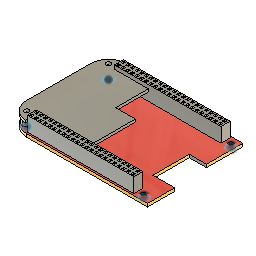
Proyektor New v3 (Autodesk Fusion 360 design; units mm, degrees)
Autodesk Fusion 360 part; units mm, degrees
sketch "Sketch1" plane through (0, 0, 0) normal (0, 0, 1) x (1, 0, 0)
  line L0 (35.75, 27.5) -> (-28.25, 27.5)
  line L1 (-38.25, 17.5) -> (-38.25, -17.5)
  line L2 (-28.25, -27.5) -> (38.25, -27.5)
  line L3 (38.25, -27.5) -> (38.25, -12.5)
  line L4 (35.75, 25.7026) -> (-34.8231, -25.0362) construction
  line L5 (-34.8231, 25.0362) -> (38.25, -27.5) construction
  line L6 (38.25, -27.5) -> (38.25, -12.5)
  line L7 (38.25, -12.5) -> (26.25, -12.5)
  line L8 (26.25, -12.5) -> (26.25, 7.5)
  line L9 (26.25, 7.5) -> (35.75, 7.5)
  line L10 (35.75, 7.5) -> (35.75, 27.5)
  arc A0 (-28.25, 27.5) -> (-38.25, 17.5) centre (-28.25, 17.5) ccw
  arc A1 (-38.25, -17.5) -> (-28.25, -27.5) centre (-28.25, -17.5) ccw
  dimension "d3" = 15
  dimension "d4" = 12
  dimension "d5" = 20
  dimension "d6" = 9.5
  dimension "d7" = 10
  constraint horizontal L0
  constraint perpendicular L0 L1
  constraint parallel L0 L2
  constraint parallel L1 L3
  constraint coincident L4 origin
  constraint coincident L5 origin
  constraint perpendicular L2 L6
  constraint perpendicular L3 L7
  constraint perpendicular L7 L8
  constraint perpendicular L3 L9
  constraint perpendicular L0 L10
  constraint tangent L0 A0
  constraint tangent L1 A0
  constraint tangent L1 A1
  constraint tangent L2 A1
  constraint equal A0 A1
  constraint coincident L10 L4.start
  constraint coincident A1 L4.end
  constraint coincident A0 L5.start
  measures "d3" distance of L2.end L3.end
  measures "d4" distance of L3.end L7.end
  measures "d5" distance of L7.end L8.end
  measures "d6" distance of L8.end L9.end
  measures "d7" radius of A0
extrude "Extrude1" add sketch "Sketch1" along normal blind 1.67 makes body 1
sketch "Sketch2" plane through (0, 0, 1.67) normal (0, 0, 1) x (-1, 0, 0)
  arc A0 (38.25, 17.5) -> (28.25, 27.5) centre (28.25, 17.5) ccw
  line L0 (28.25, 27.5) -> (-38.25, 27.5)
  line L1 (-38.25, 27.5) -> (-38.25, 12.5)
  line L2 (-38.25, 12.5) -> (-26.25, 12.5)
  line L3 (-26.25, 12.5) -> (-26.25, -7.5)
  line L4 (-26.25, -7.5) -> (-35.75, -7.5)
  line L5 (-35.75, -7.5) -> (-35.75, -27.5)
  line L6 (-35.75, -27.5) -> (28.25, -27.5)
  arc A1 (28.25, -27.5) -> (38.25, -17.5) centre (28.25, -17.5) ccw
  line L7 (38.25, -17.5) -> (38.25, 17.5)
  line L8 (-29.75, -26.5) -> (29.05, -26.5)
  line L9 (29.05, -26.5) -> (29.05, -21.5)
  line L10 (29.05, -21.5) -> (-29.75, -21.5)
  line L11 (-29.75, -21.5) -> (-29.75, -26.5)
  circle A2 centre (-32.75, -24) radius 1.25
  line L12 (-29.75, -24) -> (29.05, -24)
  line L13 (29.05, -24) -> (29.05, -26.5)
  line L14 (27.18, -24.65) -> (28.38, -24.65)
  line L15 (28.38, -24.65) -> (28.38, -25.85)
  line L16 (28.38, -25.85) -> (27.18, -25.85)
  line L17 (27.18, -25.85) -> (27.18, -24.65)
  line L18 (27.18, -24.65) -> (28.38, -25.85) construction
  line L19 (28.38, -24.65) -> (27.18, -25.85) construction
  line L20 (28.38, -22.15) -> (27.18, -22.15)
  line L21 (28.38, -23.35) -> (28.38, -22.15)
  line L22 (27.18, -22.15) -> (27.18, -23.35)
  line L23 (27.18, -23.35) -> (28.38, -23.35)
  line L24 (25.84, -25.85) -> (24.64, -25.85)
  line L25 (25.84, -24.65) -> (25.84, -25.85)
  line L26 (24.64, -25.85) -> (24.64, -24.65)
  line L27 (24.64, -24.65) -> (25.84, -24.65)
  line L28 (24.64, -23.35) -> (25.84, -23.35)
  line L29 (25.84, -23.35) -> (25.84, -22.15)
  line L30 (24.64, -22.15) -> (24.64, -23.35)
  line L31 (25.84, -22.15) -> (24.64, -22.15)
  line L32 (23.3, -25.85) -> (22.1, -25.85)
  line L33 (23.3, -24.65) -> (23.3, -25.85)
  line L34 (22.1, -25.85) -> (22.1, -24.65)
  line L35 (22.1, -24.65) -> (23.3, -24.65)
  line L36 (22.1, -23.35) -> (23.3, -23.35)
  line L37 (23.3, -23.35) -> (23.3, -22.15)
  line L38 (22.1, -22.15) -> (22.1, -23.35)
  line L39 (23.3, -22.15) -> (22.1, -22.15)
  line L40 (20.76, -25.85) -> (19.56, -25.85)
  line L41 (20.76, -24.65) -> (20.76, -25.85)
  line L42 (19.56, -25.85) -> (19.56, -24.65)
  line L43 (19.56, -24.65) -> (20.76, -24.65)
  line L44 (19.56, -23.35) -> (20.76, -23.35)
  line L45 (20.76, -23.35) -> (20.76, -22.15)
  line L46 (19.56, -22.15) -> (19.56, -23.35)
  line L47 (20.76, -22.15) -> (19.56, -22.15)
  line L48 (18.22, -25.85) -> (17.02, -25.85)
  line L49 (18.22, -24.65) -> (18.22, -25.85)
  line L50 (17.02, -25.85) -> (17.02, -24.65)
  line L51 (17.02, -24.65) -> (18.22, -24.65)
  line L52 (17.02, -23.35) -> (18.22, -23.35)
  line L53 (18.22, -23.35) -> (18.22, -22.15)
  line L54 (17.02, -22.15) -> (17.02, -23.35)
  line L55 (18.22, -22.15) -> (17.02, -22.15)
  line L56 (15.68, -25.85) -> (14.48, -25.85)
  line L57 (15.68, -24.65) -> (15.68, -25.85)
  line L58 (14.48, -25.85) -> (14.48, -24.65)
  line L59 (14.48, -24.65) -> (15.68, -24.65)
  line L60 (14.48, -23.35) -> (15.68, -23.35)
  line L61 (15.68, -23.35) -> (15.68, -22.15)
  line L62 (14.48, -22.15) -> (14.48, -23.35)
  line L63 (15.68, -22.15) -> (14.48, -22.15)
  line L64 (13.14, -25.85) -> (11.94, -25.85)
  line L65 (13.14, -24.65) -> (13.14, -25.85)
  line L66 (11.94, -25.85) -> (11.94, -24.65)
  line L67 (11.94, -24.65) -> (13.14, -24.65)
  line L68 (11.94, -23.35) -> (13.14, -23.35)
  line L69 (13.14, -23.35) -> (13.14, -22.15)
  line L70 (11.94, -22.15) -> (11.94, -23.35)
  line L71 (13.14, -22.15) -> (11.94, -22.15)
  line L72 (10.6, -25.85) -> (9.4, -25.85)
  line L73 (10.6, -24.65) -> (10.6, -25.85)
  line L74 (9.4, -25.85) -> (9.4, -24.65)
  line L75 (9.4, -24.65) -> (10.6, -24.65)
  line L76 (9.4, -23.35) -> (10.6, -23.35)
  line L77 (10.6, -23.35) -> (10.6, -22.15)
  line L78 (9.4, -22.15) -> (9.4, -23.35)
  line L79 (10.6, -22.15) -> (9.4, -22.15)
  line L80 (8.06, -25.85) -> (6.86, -25.85)
  line L81 (8.06, -24.65) -> (8.06, -25.85)
  line L82 (6.86, -25.85) -> (6.86, -24.65)
  line L83 (6.86, -24.65) -> (8.06, -24.65)
  line L84 (6.86, -23.35) -> (8.06, -23.35)
  line L85 (8.06, -23.35) -> (8.06, -22.15)
  line L86 (6.86, -22.15) -> (6.86, -23.35)
  line L87 (8.06, -22.15) -> (6.86, -22.15)
  line L88 (5.52, -25.85) -> (4.32, -25.85)
  line L89 (5.52, -24.65) -> (5.52, -25.85)
  line L90 (4.32, -25.85) -> (4.32, -24.65)
  line L91 (4.32, -24.65) -> (5.52, -24.65)
  line L92 (4.32, -23.35) -> (5.52, -23.35)
  line L93 (5.52, -23.35) -> (5.52, -22.15)
  line L94 (4.32, -22.15) -> (4.32, -23.35)
  line L95 (5.52, -22.15) -> (4.32, -22.15)
  line L96 (2.98, -25.85) -> (1.78, -25.85)
  line L97 (2.98, -24.65) -> (2.98, -25.85)
  line L98 (1.78, -25.85) -> (1.78, -24.65)
  line L99 (1.78, -24.65) -> (2.98, -24.65)
  line L100 (1.78, -23.35) -> (2.98, -23.35)
  line L101 (2.98, -23.35) -> (2.98, -22.15)
  line L102 (1.78, -22.15) -> (1.78, -23.35)
  line L103 (2.98, -22.15) -> (1.78, -22.15)
  line L104 (0.44, -25.85) -> (-0.76, -25.85)
  line L105 (0.44, -24.65) -> (0.44, -25.85)
  line L106 (-0.76, -25.85) -> (-0.76, -24.65)
  line L107 (-0.76, -24.65) -> (0.44, -24.65)
  line L108 (-0.76, -23.35) -> (0.44, -23.35)
  line L109 (0.44, -23.35) -> (0.44, -22.15)
  line L110 (-0.76, -22.15) -> (-0.76, -23.35)
  line L111 (0.44, -22.15) -> (-0.76, -22.15)
  line L112 (-2.1, -25.85) -> (-3.3, -25.85)
  line L113 (-2.1, -24.65) -> (-2.1, -25.85)
  line L114 (-3.3, -25.85) -> (-3.3, -24.65)
  line L115 (-3.3, -24.65) -> (-2.1, -24.65)
  line L116 (-3.3, -23.35) -> (-2.1, -23.35)
  line L117 (-2.1, -23.35) -> (-2.1, -22.15)
  line L118 (-3.3, -22.15) -> (-3.3, -23.35)
  line L119 (-2.1, -22.15) -> (-3.3, -22.15)
  line L120 (-4.64, -25.85) -> (-5.84, -25.85)
  line L121 (-4.64, -24.65) -> (-4.64, -25.85)
  line L122 (-5.84, -25.85) -> (-5.84, -24.65)
  line L123 (-5.84, -24.65) -> (-4.64, -24.65)
  line L124 (-5.84, -23.35) -> (-4.64, -23.35)
  line L125 (-4.64, -23.35) -> (-4.64, -22.15)
  line L126 (-5.84, -22.15) -> (-5.84, -23.35)
  line L127 (-4.64, -22.15) -> (-5.84, -22.15)
  line L128 (-7.18, -25.85) -> (-8.38, -25.85)
  line L129 (-7.18, -24.65) -> (-7.18, -25.85)
  line L130 (-8.38, -25.85) -> (-8.38, -24.65)
  line L131 (-8.38, -24.65) -> (-7.18, -24.65)
  line L132 (-8.38, -23.35) -> (-7.18, -23.35)
  line L133 (-7.18, -23.35) -> (-7.18, -22.15)
  line L134 (-8.38, -22.15) -> (-8.38, -23.35)
  line L135 (-7.18, -22.15) -> (-8.38, -22.15)
  line L136 (-9.72, -25.85) -> (-10.92, -25.85)
  line L137 (-9.72, -24.65) -> (-9.72, -25.85)
  line L138 (-10.92, -25.85) -> (-10.92, -24.65)
  line L139 (-10.92, -24.65) -> (-9.72, -24.65)
  line L140 (-10.92, -23.35) -> (-9.72, -23.35)
  line L141 (-9.72, -23.35) -> (-9.72, -22.15)
  line L142 (-10.92, -22.15) -> (-10.92, -23.35)
  line L143 (-9.72, -22.15) -> (-10.92, -22.15)
  line L144 (-12.26, -25.85) -> (-13.46, -25.85)
  line L145 (-12.26, -24.65) -> (-12.26, -25.85)
  line L146 (-13.46, -25.85) -> (-13.46, -24.65)
  line L147 (-13.46, -24.65) -> (-12.26, -24.65)
  line L148 (-13.46, -23.35) -> (-12.26, -23.35)
  line L149 (-12.26, -23.35) -> (-12.26, -22.15)
  line L150 (-13.46, -22.15) -> (-13.46, -23.35)
  line L151 (-12.26, -22.15) -> (-13.46, -22.15)
  line L152 (-14.8, -25.85) -> (-16, -25.85)
  line L153 (-14.8, -24.65) -> (-14.8, -25.85)
  line L154 (-16, -25.85) -> (-16, -24.65)
  line L155 (-16, -24.65) -> (-14.8, -24.65)
  line L156 (-16, -23.35) -> (-14.8, -23.35)
  line L157 (-14.8, -23.35) -> (-14.8, -22.15)
  line L158 (-16, -22.15) -> (-16, -23.35)
  line L159 (-14.8, -22.15) -> (-16, -22.15)
  line L160 (-17.34, -25.85) -> (-18.54, -25.85)
  line L161 (-17.34, -24.65) -> (-17.34, -25.85)
  line L162 (-18.54, -25.85) -> (-18.54, -24.65)
  line L163 (-18.54, -24.65) -> (-17.34, -24.65)
  line L164 (-18.54, -23.35) -> (-17.34, -23.35)
  line L165 (-17.34, -23.35) -> (-17.34, -22.15)
  line L166 (-18.54, -22.15) -> (-18.54, -23.35)
  line L167 (-17.34, -22.15) -> (-18.54, -22.15)
  line L168 (-19.88, -25.85) -> (-21.08, -25.85)
  line L169 (-19.88, -24.65) -> (-19.88, -25.85)
  line L170 (-21.08, -25.85) -> (-21.08, -24.65)
  line L171 (-21.08, -24.65) -> (-19.88, -24.65)
  line L172 (-21.08, -23.35) -> (-19.88, -23.35)
  line L173 (-19.88, -23.35) -> (-19.88, -22.15)
  line L174 (-21.08, -22.15) -> (-21.08, -23.35)
  line L175 (-19.88, -22.15) -> (-21.08, -22.15)
  line L176 (-22.42, -25.85) -> (-23.62, -25.85)
  line L177 (-22.42, -24.65) -> (-22.42, -25.85)
  line L178 (-23.62, -25.85) -> (-23.62, -24.65)
  line L179 (-23.62, -24.65) -> (-22.42, -24.65)
  line L180 (-23.62, -23.35) -> (-22.42, -23.35)
  line L181 (-22.42, -23.35) -> (-22.42, -22.15)
  line L182 (-23.62, -22.15) -> (-23.62, -23.35)
  line L183 (-22.42, -22.15) -> (-23.62, -22.15)
  line L184 (-24.96, -25.85) -> (-26.16, -25.85)
  line L185 (-24.96, -24.65) -> (-24.96, -25.85)
  line L186 (-26.16, -25.85) -> (-26.16, -24.65)
  line L187 (-26.16, -24.65) -> (-24.96, -24.65)
  line L188 (-26.16, -23.35) -> (-24.96, -23.35)
  line L189 (-24.96, -23.35) -> (-24.96, -22.15)
  line L190 (-26.16, -22.15) -> (-26.16, -23.35)
  line L191 (-24.96, -22.15) -> (-26.16, -22.15)
  line L192 (-27.5, -25.85) -> (-28.7, -25.85)
  line L193 (-27.5, -24.65) -> (-27.5, -25.85)
  line L194 (-28.7, -25.85) -> (-28.7, -24.65)
  line L195 (-28.7, -24.65) -> (-27.5, -24.65)
  line L196 (-28.7, -23.35) -> (-27.5, -23.35)
  line L197 (-27.5, -23.35) -> (-27.5, -22.15)
  line L198 (-28.7, -22.15) -> (-28.7, -23.35)
  line L199 (-27.5, -22.15) -> (-28.7, -22.15)
  circle A3 centre (33.25, -22.5) radius 1.25
  arc A4 (29.1, -27.4538) -> (38.24, -17.5) centre (28.25, -17.5) ccw
  line L200 (38.24, -17.5) -> (38.24, 17.5)
  arc A5 (38.24, 17.5) -> (29.1, 27.4538) centre (28.25, 17.5) ccw
  line L201 (29.1, -26.5) -> (29.1, -21.45)
  line L202 (29.1, -21.45) -> (10.24, -21.45)
  line L203 (29.1, -26.5) -> (29.1, -27.4538)
  line L204 (10.24, -21.45) -> (10.24, -3.45)
  line L205 (10.24, -3.45) -> (-0.56, -3.45)
  circle A6 centre (33.25, 22.5) radius 1.25
  line L206 (-28.7, 23.35) -> (-27.5, 23.35)
  line L207 (29.05, 21.5) -> (-29.75, 21.5)
  line L208 (29.1, 21.45) -> (-0.56, 21.45)
  line L209 (-29.75, 21.5) -> (-29.75, 26.5)
  line L210 (-22.42, 25.85) -> (-23.62, 25.85)
  line L211 (-19.88, 24.65) -> (-19.88, 25.85)
  line L212 (-21.08, 23.35) -> (-19.88, 23.35)
  line L213 (-23.62, 23.35) -> (-22.42, 23.35)
  line L214 (-24.96, 23.35) -> (-24.96, 22.15)
  line L215 (-27.5, 25.85) -> (-28.7, 25.85)
  line L216 (-22.42, 23.35) -> (-22.42, 22.15)
  line L217 (-29.75, 26.5) -> (29.05, 26.5)
  line L218 (-19.88, 25.85) -> (-21.08, 25.85)
  line L219 (-24.96, 24.65) -> (-24.96, 25.85)
  line L220 (-21.08, 22.15) -> (-21.08, 23.35)
  line L221 (-28.7, 24.65) -> (-27.5, 24.65)
  line L222 (-28.7, 22.15) -> (-28.7, 23.35)
  line L223 (-26.16, 25.85) -> (-26.16, 24.65)
  line L224 (-28.7, 25.85) -> (-28.7, 24.65)
  line L225 (-27.5, 23.35) -> (-27.5, 22.15)
  line L226 (-23.62, 25.85) -> (-23.62, 24.65)
  line L227 (-19.88, 23.35) -> (-19.88, 22.15)
  line L228 (-22.42, 22.15) -> (-23.62, 22.15)
  line L229 (-24.96, 22.15) -> (-26.16, 22.15)
  line L230 (-23.62, 24.65) -> (-22.42, 24.65)
  line L231 (-26.16, 24.65) -> (-24.96, 24.65)
  line L232 (-23.62, 22.15) -> (-23.62, 23.35)
  line L233 (-22.42, 24.65) -> (-22.42, 25.85)
  line L234 (-21.08, 24.65) -> (-19.88, 24.65)
  line L235 (-19.88, 22.15) -> (-21.08, 22.15)
  line L236 (-26.16, 22.15) -> (-26.16, 23.35)
  line L237 (-21.08, 25.85) -> (-21.08, 24.65)
  line L238 (-27.5, 24.65) -> (-27.5, 25.85)
  line L239 (-26.16, 23.35) -> (-24.96, 23.35)
  line L240 (-24.96, 25.85) -> (-26.16, 25.85)
  line L241 (-27.5, 22.15) -> (-28.7, 22.15)
  circle A7 centre (-32.75, 24) radius 1.25
  line L242 (-14.8, 23.35) -> (-14.8, 22.15)
  line L243 (-10.92, 23.35) -> (-9.72, 23.35)
  line L244 (-13.46, 24.65) -> (-12.26, 24.65)
  line L245 (-10.92, 25.85) -> (-10.92, 24.65)
  line L246 (-14.8, 24.65) -> (-14.8, 25.85)
  line L247 (8.06, 25.85) -> (6.86, 25.85)
  line L248 (-12.26, 23.35) -> (-12.26, 22.15)
  line L249 (-10.92, 24.65) -> (-9.72, 24.65)
  line L250 (-9.72, 23.35) -> (-9.72, 22.15)
  line L251 (-16, 23.35) -> (-14.8, 23.35)
  line L252 (-12.26, 25.85) -> (-13.46, 25.85)
  line L253 (-16, 24.65) -> (-14.8, 24.65)
  line L254 (-13.46, 25.85) -> (-13.46, 24.65)
  line L255 (-12.26, 24.65) -> (-12.26, 25.85)
  line L256 (-9.72, 24.65) -> (-9.72, 25.85)
  line L257 (1.78, 23.35) -> (2.98, 23.35)
  line L258 (-13.46, 23.35) -> (-12.26, 23.35)
  line L259 (-10.92, 22.15) -> (-10.92, 23.35)
  line L260 (-16, 22.15) -> (-16, 23.35)
  line L261 (-16, 25.85) -> (-16, 24.65)
  line L262 (-13.46, 22.15) -> (-13.46, 23.35)
  line L263 (-14.8, 25.85) -> (-16, 25.85)
  line L264 (-8.38, 25.85) -> (-8.38, 24.65)
  line L265 (1.78, 22.15) -> (1.78, 23.35)
  line L266 (-3.3, 25.85) -> (-3.3, 24.65)
  line L267 (-0.76, 22.15) -> (-0.76, 23.35)
  line L268 (22.1, 24.65) -> (23.3, 24.65)
  line L269 (20.76, 23.35) -> (20.76, 22.15)
  line L270 (28.38, 23.35) -> (28.38, 22.15)
  line L271 (9.4, 22.15) -> (9.4, 23.35)
  line L272 (10.6, 23.35) -> (10.6, 22.15)
  line L273 (22.1, 23.35) -> (23.3, 23.35)
  line L274 (23.3, 23.35) -> (23.3, 22.15)
  line L275 (9.4, 25.85) -> (9.4, 24.65)
  line L276 (25.84, 24.65) -> (25.84, 25.85)
  line L277 (25.84, 25.85) -> (24.64, 25.85)
  line L278 (-8.38, 24.65) -> (-7.18, 24.65)
  line L279 (6.86, 22.15) -> (6.86, 23.35)
  line L280 (28.38, 24.65) -> (28.38, 25.85)
  line L281 (0.44, 25.85) -> (-0.76, 25.85)
  line L282 (24.64, 22.15) -> (24.64, 23.35)
  line L283 (4.32, 22.15) -> (4.32, 23.35)
  line L284 (22.1, 25.85) -> (22.1, 24.65)
  line L285 (1.78, 25.85) -> (1.78, 24.65)
  line L286 (6.86, 25.85) -> (6.86, 24.65)
  line L287 (4.32, 25.85) -> (4.32, 24.65)
  line L288 (-8.38, 22.15) -> (-8.38, 23.35)
  line L289 (24.64, 24.65) -> (25.84, 24.65)
  line L290 (19.56, 22.15) -> (19.56, 23.35)
  line L291 (20.76, 25.85) -> (19.56, 25.85)
  line L292 (27.18, 22.15) -> (27.18, 23.35)
  line L293 (-9.72, 25.85) -> (-10.92, 25.85)
  line L294 (19.56, 23.35) -> (20.76, 23.35)
  line L295 (-2.1, 24.65) -> (-2.1, 25.85)
  line L296 (28.38, 25.85) -> (27.18, 25.85)
  line L297 (-4.64, 25.85) -> (-5.84, 25.85)
  line L298 (-17.34, 25.85) -> (-18.54, 25.85)
  line L299 (22.1, 22.15) -> (22.1, 23.35)
  line L300 (27.18, 23.35) -> (28.38, 23.35)
  line L301 (25.84, 23.35) -> (25.84, 22.15)
  line L302 (9.4, 23.35) -> (10.6, 23.35)
  line L303 (-18.54, 23.35) -> (-17.34, 23.35)
  line L304 (10.6, 25.85) -> (9.4, 25.85)
  line L305 (-4.64, 23.35) -> (-4.64, 22.15)
  line L306 (-3.3, 23.35) -> (-2.1, 23.35)
  line L307 (2.98, 23.35) -> (2.98, 22.15)
  line L308 (2.98, 25.85) -> (1.78, 25.85)
  line L309 (-18.54, 25.85) -> (-18.54, 24.65)
  line L310 (-0.76, 23.35) -> (0.44, 23.35)
  line L311 (-2.1, 25.85) -> (-3.3, 25.85)
  line L312 (19.56, 24.65) -> (20.76, 24.65)
  line L313 (4.32, 24.65) -> (5.52, 24.65)
  line L314 (8.06, 24.65) -> (8.06, 25.85)
  line L315 (19.56, 25.85) -> (19.56, 24.65)
  line L316 (-4.64, 24.65) -> (-4.64, 25.85)
  line L317 (27.18, 24.65) -> (28.38, 24.65)
  line L318 (1.78, 24.65) -> (2.98, 24.65)
  line L319 (0.44, 24.65) -> (0.44, 25.85)
  line L320 (23.3, 25.85) -> (22.1, 25.85)
  line L321 (9.4, 24.65) -> (10.6, 24.65)
  line L322 (24.64, 25.85) -> (24.64, 24.65)
  line L323 (-0.76, 24.65) -> (0.44, 24.65)
  line L324 (-3.3, 24.65) -> (-2.1, 24.65)
  line L325 (-17.34, 23.35) -> (-17.34, 22.15)
  line L326 (-7.18, 25.85) -> (-8.38, 25.85)
  line L327 (-5.84, 24.65) -> (-4.64, 24.65)
  line L328 (23.3, 24.65) -> (23.3, 25.85)
  line L329 (27.18, 25.85) -> (27.18, 24.65)
  line L330 (5.52, 23.35) -> (5.52, 22.15)
  line L331 (-3.3, 22.15) -> (-3.3, 23.35)
  line L332 (6.86, 23.35) -> (8.06, 23.35)
  line L333 (0.44, 23.35) -> (0.44, 22.15)
  line L334 (-5.84, 22.15) -> (-5.84, 23.35)
  line L335 (10.6, 24.65) -> (10.6, 25.85)
  line L336 (24.64, 23.35) -> (25.84, 23.35)
  line L337 (-7.18, 23.35) -> (-7.18, 22.15)
  line L338 (-0.76, 25.85) -> (-0.76, 24.65)
  line L339 (5.52, 25.85) -> (4.32, 25.85)
  line L340 (20.76, 24.65) -> (20.76, 25.85)
  line L341 (-5.84, 25.85) -> (-5.84, 24.65)
  line L342 (-8.38, 23.35) -> (-7.18, 23.35)
  line L343 (2.98, 24.65) -> (2.98, 25.85)
  line L344 (-5.84, 23.35) -> (-4.64, 23.35)
  line L345 (-18.54, 22.15) -> (-18.54, 23.35)
  line L346 (-17.34, 24.65) -> (-17.34, 25.85)
  line L347 (-2.1, 23.35) -> (-2.1, 22.15)
  line L348 (-18.54, 24.65) -> (-17.34, 24.65)
  line L349 (-7.18, 24.65) -> (-7.18, 25.85)
  line L350 (14.48, 24.65) -> (15.68, 24.65)
  line L351 (5.52, 24.65) -> (5.52, 25.85)
  line L352 (11.94, 22.15) -> (11.94, 23.35)
  line L353 (17.02, 23.35) -> (18.22, 23.35)
  line L354 (15.68, 25.85) -> (14.48, 25.85)
  line L355 (13.14, 23.35) -> (13.14, 22.15)
  line L356 (18.22, 25.85) -> (17.02, 25.85)
  line L357 (14.48, 25.85) -> (14.48, 24.65)
  line L358 (17.02, 24.65) -> (18.22, 24.65)
  line L359 (17.02, 22.15) -> (17.02, 23.35)
  line L360 (18.22, 23.35) -> (18.22, 22.15)
  line L361 (4.32, 23.35) -> (5.52, 23.35)
  line L362 (14.48, 23.35) -> (15.68, 23.35)
  line L363 (13.14, 24.65) -> (13.14, 25.85)
  line L364 (11.94, 25.85) -> (11.94, 24.65)
  line L365 (18.22, 24.65) -> (18.22, 25.85)
  line L366 (14.48, 22.15) -> (14.48, 23.35)
  line L367 (15.68, 23.35) -> (15.68, 22.15)
  line L368 (8.06, 23.35) -> (8.06, 22.15)
  line L369 (17.02, 25.85) -> (17.02, 24.65)
  line L370 (6.86, 24.65) -> (8.06, 24.65)
  line L371 (13.14, 25.85) -> (11.94, 25.85)
  line L372 (11.94, 23.35) -> (13.14, 23.35)
  line L373 (11.94, 24.65) -> (13.14, 24.65)
  line L374 (15.68, 24.65) -> (15.68, 25.85)
  line L375 (28.38, 22.15) -> (27.18, 22.15)
  line L376 (25.84, 22.15) -> (24.64, 22.15)
  line L377 (23.3, 22.15) -> (22.1, 22.15)
  line L378 (20.76, 22.15) -> (19.56, 22.15)
  line L379 (18.22, 22.15) -> (17.02, 22.15)
  line L380 (15.68, 22.15) -> (14.48, 22.15)
  line L381 (13.14, 22.15) -> (11.94, 22.15)
  line L382 (10.6, 22.15) -> (9.4, 22.15)
  line L383 (8.06, 22.15) -> (6.86, 22.15)
  line L384 (5.52, 22.15) -> (4.32, 22.15)
  line L385 (2.98, 22.15) -> (1.78, 22.15)
  line L386 (0.44, 22.15) -> (-0.76, 22.15)
  line L387 (-2.1, 22.15) -> (-3.3, 22.15)
  line L388 (-4.64, 22.15) -> (-5.84, 22.15)
  line L389 (-7.18, 22.15) -> (-8.38, 22.15)
  line L390 (-9.72, 22.15) -> (-10.92, 22.15)
  line L391 (-12.26, 22.15) -> (-13.46, 22.15)
  line L392 (-14.8, 22.15) -> (-16, 22.15)
  line L393 (-17.34, 22.15) -> (-18.54, 22.15)
  line L394 (29.05, 21.5) -> (29.05, 26.5)
  line L395 (-0.56, -3.45) -> (-0.56, 21.45)
  line L396 (29.1, 21.45) -> (29.1, 27.4538)
  line L397 (27.58, 25.05) -> (27.98, 25.05)
  line L398 (27.98, 25.05) -> (27.98, 25.45)
  line L399 (27.98, 25.45) -> (27.58, 25.45)
  line L400 (27.58, 25.45) -> (27.58, 25.05)
  line L401 (29.05, 24) -> (27.6, 24)
  line L402 (27.98, 22.95) -> (27.98, 22.55)
  line L403 (27.58, 22.95) -> (27.98, 22.95)
  line L404 (27.58, 22.55) -> (27.58, 22.95)
  line L405 (27.98, 22.55) -> (27.58, 22.55)
  line L406 (25.04, 25.45) -> (25.04, 25.05)
  line L407 (25.44, 25.05) -> (25.44, 25.45)
  line L408 (25.04, 25.05) -> (25.44, 25.05)
  line L409 (25.44, 25.45) -> (25.04, 25.45)
  line L410 (25.04, 22.95) -> (25.44, 22.95)
  line L411 (25.44, 22.55) -> (25.04, 22.55)
  line L412 (25.44, 22.95) -> (25.44, 22.55)
  line L413 (25.04, 22.55) -> (25.04, 22.95)
  line L414 (22.5, 25.45) -> (22.5, 25.05)
  line L415 (22.9, 25.05) -> (22.9, 25.45)
  line L416 (22.5, 25.05) -> (22.9, 25.05)
  line L417 (22.9, 25.45) -> (22.5, 25.45)
  line L418 (22.5, 22.95) -> (22.9, 22.95)
  line L419 (22.9, 22.55) -> (22.5, 22.55)
  line L420 (22.9, 22.95) -> (22.9, 22.55)
  line L421 (22.5, 22.55) -> (22.5, 22.95)
  line L422 (19.96, 25.45) -> (19.96, 25.05)
  line L423 (20.36, 25.05) -> (20.36, 25.45)
  line L424 (19.96, 25.05) -> (20.36, 25.05)
  line L425 (20.36, 25.45) -> (19.96, 25.45)
  line L426 (19.96, 22.95) -> (20.36, 22.95)
  line L427 (20.36, 22.55) -> (19.96, 22.55)
  line L428 (20.36, 22.95) -> (20.36, 22.55)
  line L429 (19.96, 22.55) -> (19.96, 22.95)
  line L430 (17.42, 25.45) -> (17.42, 25.05)
  line L431 (17.82, 25.05) -> (17.82, 25.45)
  line L432 (17.42, 25.05) -> (17.82, 25.05)
  line L433 (17.82, 25.45) -> (17.42, 25.45)
  line L434 (17.42, 22.95) -> (17.82, 22.95)
  line L435 (17.82, 22.55) -> (17.42, 22.55)
  line L436 (17.82, 22.95) -> (17.82, 22.55)
  line L437 (17.42, 22.55) -> (17.42, 22.95)
  line L438 (14.88, 25.45) -> (14.88, 25.05)
  line L439 (15.28, 25.05) -> (15.28, 25.45)
  line L440 (14.88, 25.05) -> (15.28, 25.05)
  line L441 (15.28, 25.45) -> (14.88, 25.45)
  line L442 (14.88, 22.95) -> (15.28, 22.95)
  line L443 (15.28, 22.55) -> (14.88, 22.55)
  line L444 (15.28, 22.95) -> (15.28, 22.55)
  line L445 (14.88, 22.55) -> (14.88, 22.95)
  line L446 (12.34, 25.45) -> (12.34, 25.05)
  line L447 (12.74, 25.05) -> (12.74, 25.45)
  line L448 (12.34, 25.05) -> (12.74, 25.05)
  line L449 (12.74, 25.45) -> (12.34, 25.45)
  line L450 (12.34, 22.95) -> (12.74, 22.95)
  line L451 (12.74, 22.55) -> (12.34, 22.55)
  line L452 (12.74, 22.95) -> (12.74, 22.55)
  line L453 (12.34, 22.55) -> (12.34, 22.95)
  line L454 (9.8, 25.45) -> (9.8, 25.05)
  line L455 (10.2, 25.05) -> (10.2, 25.45)
  line L456 (9.8, 25.05) -> (10.2, 25.05)
  line L457 (10.2, 25.45) -> (9.8, 25.45)
  line L458 (9.8, 22.95) -> (10.2, 22.95)
  line L459 (10.2, 22.55) -> (9.8, 22.55)
  line L460 (10.2, 22.95) -> (10.2, 22.55)
  line L461 (9.8, 22.55) -> (9.8, 22.95)
  line L462 (7.26, 25.45) -> (7.26, 25.05)
  line L463 (7.66, 25.05) -> (7.66, 25.45)
  line L464 (7.26, 25.05) -> (7.66, 25.05)
  line L465 (7.66, 25.45) -> (7.26, 25.45)
  line L466 (7.26, 22.95) -> (7.66, 22.95)
  line L467 (7.66, 22.55) -> (7.26, 22.55)
  line L468 (7.66, 22.95) -> (7.66, 22.55)
  line L469 (7.26, 22.55) -> (7.26, 22.95)
  line L470 (4.72, 25.45) -> (4.72, 25.05)
  line L471 (5.12, 25.05) -> (5.12, 25.45)
  line L472 (4.72, 25.05) -> (5.12, 25.05)
  line L473 (5.12, 25.45) -> (4.72, 25.45)
  line L474 (4.72, 22.95) -> (5.12, 22.95)
  line L475 (5.12, 22.55) -> (4.72, 22.55)
  line L476 (5.12, 22.95) -> (5.12, 22.55)
  line L477 (4.72, 22.55) -> (4.72, 22.95)
  line L478 (2.18, 25.45) -> (2.18, 25.05)
  line L479 (2.58, 25.05) -> (2.58, 25.45)
  line L480 (2.18, 25.05) -> (2.58, 25.05)
  line L481 (2.58, 25.45) -> (2.18, 25.45)
  line L482 (2.18, 22.95) -> (2.58, 22.95)
  line L483 (2.58, 22.55) -> (2.18, 22.55)
  line L484 (2.58, 22.95) -> (2.58, 22.55)
  line L485 (2.18, 22.55) -> (2.18, 22.95)
  line L486 (-0.36, 25.45) -> (-0.36, 25.05)
  line L487 (0.04, 25.05) -> (0.04, 25.45)
  line L488 (-0.36, 25.05) -> (0.04, 25.05)
  line L489 (0.04, 25.45) -> (-0.36, 25.45)
  line L490 (-0.36, 22.95) -> (0.04, 22.95)
  line L491 (0.04, 22.55) -> (-0.36, 22.55)
  line L492 (0.04, 22.95) -> (0.04, 22.55)
  line L493 (-0.36, 22.55) -> (-0.36, 22.95)
  line L494 (-2.9, 25.45) -> (-2.9, 25.05)
  line L495 (-2.5, 25.05) -> (-2.5, 25.45)
  line L496 (-2.9, 25.05) -> (-2.5, 25.05)
  line L497 (-2.5, 25.45) -> (-2.9, 25.45)
  line L498 (-2.9, 22.95) -> (-2.5, 22.95)
  line L499 (-2.5, 22.55) -> (-2.9, 22.55)
  line L500 (-2.5, 22.95) -> (-2.5, 22.55)
  line L501 (-2.9, 22.55) -> (-2.9, 22.95)
  line L502 (-5.44, 25.45) -> (-5.44, 25.05)
  line L503 (-5.04, 25.05) -> (-5.04, 25.45)
  line L504 (-5.44, 25.05) -> (-5.04, 25.05)
  line L505 (-5.04, 25.45) -> (-5.44, 25.45)
  line L506 (-5.44, 22.95) -> (-5.04, 22.95)
  line L507 (-5.04, 22.55) -> (-5.44, 22.55)
  line L508 (-5.04, 22.95) -> (-5.04, 22.55)
  line L509 (-5.44, 22.55) -> (-5.44, 22.95)
  line L510 (-7.98, 25.45) -> (-7.98, 25.05)
  line L511 (-7.58, 25.05) -> (-7.58, 25.45)
  line L512 (-7.98, 25.05) -> (-7.58, 25.05)
  line L513 (-7.58, 25.45) -> (-7.98, 25.45)
  line L514 (-7.98, 22.95) -> (-7.58, 22.95)
  line L515 (-7.58, 22.55) -> (-7.98, 22.55)
  line L516 (-7.58, 22.95) -> (-7.58, 22.55)
  line L517 (-7.98, 22.55) -> (-7.98, 22.95)
  line L518 (-10.52, 25.45) -> (-10.52, 25.05)
  line L519 (-10.12, 25.05) -> (-10.12, 25.45)
  line L520 (-10.52, 25.05) -> (-10.12, 25.05)
  line L521 (-10.12, 25.45) -> (-10.52, 25.45)
  line L522 (-10.52, 22.95) -> (-10.12, 22.95)
  line L523 (-10.12, 22.55) -> (-10.52, 22.55)
  line L524 (-10.12, 22.95) -> (-10.12, 22.55)
  line L525 (-10.52, 22.55) -> (-10.52, 22.95)
  line L526 (-13.06, 25.45) -> (-13.06, 25.05)
  line L527 (-12.66, 25.05) -> (-12.66, 25.45)
  line L528 (-13.06, 25.05) -> (-12.66, 25.05)
  line L529 (-12.66, 25.45) -> (-13.06, 25.45)
  line L530 (-13.06, 22.95) -> (-12.66, 22.95)
  line L531 (-12.66, 22.55) -> (-13.06, 22.55)
  line L532 (-12.66, 22.95) -> (-12.66, 22.55)
  line L533 (-13.06, 22.55) -> (-13.06, 22.95)
  line L534 (-15.6, 25.45) -> (-15.6, 25.05)
  line L535 (-15.2, 25.05) -> (-15.2, 25.45)
  line L536 (-15.6, 25.05) -> (-15.2, 25.05)
  line L537 (-15.2, 25.45) -> (-15.6, 25.45)
  line L538 (-15.6, 22.95) -> (-15.2, 22.95)
  line L539 (-15.2, 22.55) -> (-15.6, 22.55)
  line L540 (-15.2, 22.95) -> (-15.2, 22.55)
  line L541 (-15.6, 22.55) -> (-15.6, 22.95)
  line L542 (-18.14, 25.45) -> (-18.14, 25.05)
  line L543 (-17.74, 25.05) -> (-17.74, 25.45)
  line L544 (-18.14, 25.05) -> (-17.74, 25.05)
  line L545 (-17.74, 25.45) -> (-18.14, 25.45)
  line L546 (-18.14, 22.95) -> (-17.74, 22.95)
  line L547 (-17.74, 22.55) -> (-18.14, 22.55)
  line L548 (-17.74, 22.95) -> (-17.74, 22.55)
  line L549 (-18.14, 22.55) -> (-18.14, 22.95)
  line L550 (-20.68, 25.45) -> (-20.68, 25.05)
  line L551 (-20.28, 25.05) -> (-20.28, 25.45)
  line L552 (-20.68, 25.05) -> (-20.28, 25.05)
  line L553 (-20.28, 25.45) -> (-20.68, 25.45)
  line L554 (-20.68, 22.95) -> (-20.28, 22.95)
  line L555 (-20.28, 22.55) -> (-20.68, 22.55)
  line L556 (-20.28, 22.95) -> (-20.28, 22.55)
  line L557 (-20.68, 22.55) -> (-20.68, 22.95)
  line L558 (-23.22, 25.45) -> (-23.22, 25.05)
  line L559 (-22.82, 25.05) -> (-22.82, 25.45)
  line L560 (-23.22, 25.05) -> (-22.82, 25.05)
  line L561 (-22.82, 25.45) -> (-23.22, 25.45)
  line L562 (-23.22, 22.95) -> (-22.82, 22.95)
  line L563 (-22.82, 22.55) -> (-23.22, 22.55)
  line L564 (-22.82, 22.95) -> (-22.82, 22.55)
  line L565 (-23.22, 22.55) -> (-23.22, 22.95)
  line L566 (-25.76, 25.45) -> (-25.76, 25.05)
  line L567 (-25.36, 25.05) -> (-25.36, 25.45)
  line L568 (-25.76, 25.05) -> (-25.36, 25.05)
  line L569 (-25.36, 25.45) -> (-25.76, 25.45)
  line L570 (-25.76, 22.95) -> (-25.36, 22.95)
  line L571 (-25.36, 22.55) -> (-25.76, 22.55)
  line L572 (-25.36, 22.95) -> (-25.36, 22.55)
  line L573 (-25.76, 22.55) -> (-25.76, 22.95)
  line L574 (-28.3, 25.45) -> (-28.3, 25.05)
  line L575 (-27.9, 25.05) -> (-27.9, 25.45)
  line L576 (-28.3, 25.05) -> (-27.9, 25.05)
  line L577 (-27.9, 25.45) -> (-28.3, 25.45)
  line L578 (-28.3, 22.95) -> (-27.9, 22.95)
  line L579 (-27.9, 22.55) -> (-28.3, 22.55)
  line L580 (-27.9, 22.95) -> (-27.9, 22.55)
  line L581 (-28.3, 22.55) -> (-28.3, 22.95)
  line L582 (27.58, -22.95) -> (27.98, -22.95)
  line L583 (27.98, -22.95) -> (27.98, -22.55)
  line L584 (27.98, -22.55) -> (27.58, -22.55)
  line L585 (27.58, -22.55) -> (27.58, -22.95)
  line L586 (27.58, -25.45) -> (27.58, -25.05)
  line L587 (27.58, -25.05) -> (27.98, -25.05)
  line L588 (27.98, -25.05) -> (27.98, -25.45)
  line L589 (27.98, -25.45) -> (27.58, -25.45)
  line L590 (25.04, -22.95) -> (25.44, -22.95)
  line L591 (25.44, -22.95) -> (25.44, -22.55)
  line L592 (25.44, -22.55) -> (25.04, -22.55)
  line L593 (25.04, -22.55) -> (25.04, -22.95)
  line L594 (25.44, -25.45) -> (25.04, -25.45)
  line L595 (25.44, -25.05) -> (25.44, -25.45)
  line L596 (25.04, -25.05) -> (25.44, -25.05)
  line L597 (25.04, -25.45) -> (25.04, -25.05)
  line L598 (22.5, -22.95) -> (22.9, -22.95)
  line L599 (22.9, -22.95) -> (22.9, -22.55)
  line L600 (22.9, -22.55) -> (22.5, -22.55)
  line L601 (22.5, -22.55) -> (22.5, -22.95)
  line L602 (22.9, -25.45) -> (22.5, -25.45)
  line L603 (22.9, -25.05) -> (22.9, -25.45)
  line L604 (22.5, -25.05) -> (22.9, -25.05)
  line L605 (22.5, -25.45) -> (22.5, -25.05)
  line L606 (19.96, -22.95) -> (20.36, -22.95)
  line L607 (20.36, -22.95) -> (20.36, -22.55)
  line L608 (20.36, -22.55) -> (19.96, -22.55)
  line L609 (19.96, -22.55) -> (19.96, -22.95)
  line L610 (20.36, -25.45) -> (19.96, -25.45)
  line L611 (20.36, -25.05) -> (20.36, -25.45)
  line L612 (19.96, -25.05) -> (20.36, -25.05)
  line L613 (19.96, -25.45) -> (19.96, -25.05)
  line L614 (17.42, -22.95) -> (17.82, -22.95)
  line L615 (17.82, -22.95) -> (17.82, -22.55)
  line L616 (17.82, -22.55) -> (17.42, -22.55)
  line L617 (17.42, -22.55) -> (17.42, -22.95)
  line L618 (17.82, -25.45) -> (17.42, -25.45)
  line L619 (17.82, -25.05) -> (17.82, -25.45)
  line L620 (17.42, -25.05) -> (17.82, -25.05)
  line L621 (17.42, -25.45) -> (17.42, -25.05)
  line L622 (14.88, -22.95) -> (15.28, -22.95)
  line L623 (15.28, -22.95) -> (15.28, -22.55)
  line L624 (15.28, -22.55) -> (14.88, -22.55)
  line L625 (14.88, -22.55) -> (14.88, -22.95)
  line L626 (15.28, -25.45) -> (14.88, -25.45)
  line L627 (15.28, -25.05) -> (15.28, -25.45)
  line L628 (14.88, -25.05) -> (15.28, -25.05)
  line L629 (14.88, -25.45) -> (14.88, -25.05)
  line L630 (12.34, -22.95) -> (12.74, -22.95)
  line L631 (12.74, -22.95) -> (12.74, -22.55)
  line L632 (12.74, -22.55) -> (12.34, -22.55)
  line L633 (12.34, -22.55) -> (12.34, -22.95)
  line L634 (12.74, -25.45) -> (12.34, -25.45)
  line L635 (12.74, -25.05) -> (12.74, -25.45)
  line L636 (12.34, -25.05) -> (12.74, -25.05)
  line L637 (12.34, -25.45) -> (12.34, -25.05)
  line L638 (9.8, -22.95) -> (10.2, -22.95)
  line L639 (10.2, -22.95) -> (10.2, -22.55)
  line L640 (10.2, -22.55) -> (9.8, -22.55)
  line L641 (9.8, -22.55) -> (9.8, -22.95)
  line L642 (10.2, -25.45) -> (9.8, -25.45)
  line L643 (10.2, -25.05) -> (10.2, -25.45)
  line L644 (9.8, -25.05) -> (10.2, -25.05)
  line L645 (9.8, -25.45) -> (9.8, -25.05)
  line L646 (7.26, -22.95) -> (7.66, -22.95)
  line L647 (7.66, -22.95) -> (7.66, -22.55)
  line L648 (7.66, -22.55) -> (7.26, -22.55)
  line L649 (7.26, -22.55) -> (7.26, -22.95)
  line L650 (7.66, -25.45) -> (7.26, -25.45)
  line L651 (7.66, -25.05) -> (7.66, -25.45)
  line L652 (7.26, -25.05) -> (7.66, -25.05)
  line L653 (7.26, -25.45) -> (7.26, -25.05)
  line L654 (4.72, -22.95) -> (5.12, -22.95)
  line L655 (5.12, -22.95) -> (5.12, -22.55)
  line L656 (5.12, -22.55) -> (4.72, -22.55)
  line L657 (4.72, -22.55) -> (4.72, -22.95)
  line L658 (5.12, -25.45) -> (4.72, -25.45)
  line L659 (5.12, -25.05) -> (5.12, -25.45)
  line L660 (4.72, -25.05) -> (5.12, -25.05)
  line L661 (4.72, -25.45) -> (4.72, -25.05)
  line L662 (2.18, -22.95) -> (2.58, -22.95)
  line L663 (2.58, -22.95) -> (2.58, -22.55)
  line L664 (2.58, -22.55) -> (2.18, -22.55)
  line L665 (2.18, -22.55) -> (2.18, -22.95)
  line L666 (2.58, -25.45) -> (2.18, -25.45)
  line L667 (2.58, -25.05) -> (2.58, -25.45)
  line L668 (2.18, -25.05) -> (2.58, -25.05)
  line L669 (2.18, -25.45) -> (2.18, -25.05)
  line L670 (-0.36, -22.95) -> (0.04, -22.95)
  line L671 (0.04, -22.95) -> (0.04, -22.55)
  line L672 (0.04, -22.55) -> (-0.36, -22.55)
  line L673 (-0.36, -22.55) -> (-0.36, -22.95)
  line L674 (0.04, -25.45) -> (-0.36, -25.45)
  line L675 (0.04, -25.05) -> (0.04, -25.45)
  line L676 (-0.36, -25.05) -> (0.04, -25.05)
  line L677 (-0.36, -25.45) -> (-0.36, -25.05)
  line L678 (-2.9, -22.95) -> (-2.5, -22.95)
  line L679 (-2.5, -22.95) -> (-2.5, -22.55)
  line L680 (-2.5, -22.55) -> (-2.9, -22.55)
  line L681 (-2.9, -22.55) -> (-2.9, -22.95)
  line L682 (-2.5, -25.45) -> (-2.9, -25.45)
  line L683 (-2.5, -25.05) -> (-2.5, -25.45)
  line L684 (-2.9, -25.05) -> (-2.5, -25.05)
  line L685 (-2.9, -25.45) -> (-2.9, -25.05)
  line L686 (-5.44, -22.95) -> (-5.04, -22.95)
  line L687 (-5.04, -22.95) -> (-5.04, -22.55)
  line L688 (-5.04, -22.55) -> (-5.44, -22.55)
  line L689 (-5.44, -22.55) -> (-5.44, -22.95)
  line L690 (-5.04, -25.45) -> (-5.44, -25.45)
  line L691 (-5.04, -25.05) -> (-5.04, -25.45)
  line L692 (-5.44, -25.05) -> (-5.04, -25.05)
  line L693 (-5.44, -25.45) -> (-5.44, -25.05)
  line L694 (-7.98, -22.95) -> (-7.58, -22.95)
  line L695 (-7.58, -22.95) -> (-7.58, -22.55)
  line L696 (-7.58, -22.55) -> (-7.98, -22.55)
  line L697 (-7.98, -22.55) -> (-7.98, -22.95)
  line L698 (-7.58, -25.45) -> (-7.98, -25.45)
  line L699 (-7.58, -25.05) -> (-7.58, -25.45)
  line L700 (-7.98, -25.05) -> (-7.58, -25.05)
  line L701 (-7.98, -25.45) -> (-7.98, -25.05)
  line L702 (-10.52, -22.95) -> (-10.12, -22.95)
  line L703 (-10.12, -22.95) -> (-10.12, -22.55)
  line L704 (-10.12, -22.55) -> (-10.52, -22.55)
  line L705 (-10.52, -22.55) -> (-10.52, -22.95)
  line L706 (-10.12, -25.45) -> (-10.52, -25.45)
  line L707 (-10.12, -25.05) -> (-10.12, -25.45)
  line L708 (-10.52, -25.05) -> (-10.12, -25.05)
  line L709 (-10.52, -25.45) -> (-10.52, -25.05)
  line L710 (-13.06, -22.95) -> (-12.66, -22.95)
  line L711 (-12.66, -22.95) -> (-12.66, -22.55)
  line L712 (-12.66, -22.55) -> (-13.06, -22.55)
  line L713 (-13.06, -22.55) -> (-13.06, -22.95)
  line L714 (-12.66, -25.45) -> (-13.06, -25.45)
  line L715 (-12.66, -25.05) -> (-12.66, -25.45)
  line L716 (-13.06, -25.05) -> (-12.66, -25.05)
  line L717 (-13.06, -25.45) -> (-13.06, -25.05)
  line L718 (-15.6, -22.95) -> (-15.2, -22.95)
  line L719 (-15.2, -22.95) -> (-15.2, -22.55)
  line L720 (-15.2, -22.55) -> (-15.6, -22.55)
  line L721 (-15.6, -22.55) -> (-15.6, -22.95)
  line L722 (-15.2, -25.45) -> (-15.6, -25.45)
  line L723 (-15.2, -25.05) -> (-15.2, -25.45)
  line L724 (-15.6, -25.05) -> (-15.2, -25.05)
  line L725 (-15.6, -25.45) -> (-15.6, -25.05)
  line L726 (-18.14, -22.95) -> (-17.74, -22.95)
  line L727 (-17.74, -22.95) -> (-17.74, -22.55)
  line L728 (-17.74, -22.55) -> (-18.14, -22.55)
  line L729 (-18.14, -22.55) -> (-18.14, -22.95)
  line L730 (-17.74, -25.45) -> (-18.14, -25.45)
  line L731 (-17.74, -25.05) -> (-17.74, -25.45)
  line L732 (-18.14, -25.05) -> (-17.74, -25.05)
  line L733 (-18.14, -25.45) -> (-18.14, -25.05)
  line L734 (-20.68, -22.95) -> (-20.28, -22.95)
  line L735 (-20.28, -22.95) -> (-20.28, -22.55)
  line L736 (-20.28, -22.55) -> (-20.68, -22.55)
  line L737 (-20.68, -22.55) -> (-20.68, -22.95)
  line L738 (-20.28, -25.45) -> (-20.68, -25.45)
  line L739 (-20.28, -25.05) -> (-20.28, -25.45)
  line L740 (-20.68, -25.05) -> (-20.28, -25.05)
  line L741 (-20.68, -25.45) -> (-20.68, -25.05)
  line L742 (-23.22, -22.95) -> (-22.82, -22.95)
  line L743 (-22.82, -22.95) -> (-22.82, -22.55)
  line L744 (-22.82, -22.55) -> (-23.22, -22.55)
  line L745 (-23.22, -22.55) -> (-23.22, -22.95)
  line L746 (-22.82, -25.45) -> (-23.22, -25.45)
  line L747 (-22.82, -25.05) -> (-22.82, -25.45)
  line L748 (-23.22, -25.05) -> (-22.82, -25.05)
  line L749 (-23.22, -25.45) -> (-23.22, -25.05)
  line L750 (-25.76, -22.95) -> (-25.36, -22.95)
  line L751 (-25.36, -22.95) -> (-25.36, -22.55)
  line L752 (-25.36, -22.55) -> (-25.76, -22.55)
  line L753 (-25.76, -22.55) -> (-25.76, -22.95)
  line L754 (-25.36, -25.45) -> (-25.76, -25.45)
  line L755 (-25.36, -25.05) -> (-25.36, -25.45)
  line L756 (-25.76, -25.05) -> (-25.36, -25.05)
  line L757 (-25.76, -25.45) -> (-25.76, -25.05)
  line L758 (-28.3, -22.95) -> (-27.9, -22.95)
  line L759 (-27.9, -22.95) -> (-27.9, -22.55)
  line L760 (-27.9, -22.55) -> (-28.3, -22.55)
  line L761 (-28.3, -22.55) -> (-28.3, -22.95)
  line L762 (-27.9, -25.45) -> (-28.3, -25.45)
  line L763 (-27.9, -25.05) -> (-27.9, -25.45)
  line L764 (-28.3, -25.05) -> (-27.9, -25.05)
  line L765 (-28.3, -25.45) -> (-28.3, -25.05)
  point P0 (27.78, -25.25)
  point P1 (-29.75, 24)
  point P2 (27.78, 25.25)
  point P3 (29.05, 24)
  point P4 (27.78, 22.75)
  point P5 (25.24, 25.25)
  point P6 (25.24, 22.75)
  point P7 (22.7, 25.25)
  point P8 (22.7, 22.75)
  point P9 (20.16, 25.25)
  point P10 (20.16, 22.75)
  point P11 (17.62, 25.25)
  point P12 (17.62, 22.75)
  point P13 (15.08, 25.25)
  point P14 (15.08, 22.75)
  point P15 (12.54, 25.25)
  point P16 (12.54, 22.75)
  point P17 (10, 25.25)
  point P18 (10, 22.75)
  point P19 (7.46, 25.25)
  point P20 (7.46, 22.75)
  point P21 (4.92, 25.25)
  point P22 (4.92, 22.75)
  point P23 (2.38, 25.25)
  point P24 (2.38, 22.75)
  point P25 (-0.16, 25.25)
  point P26 (-0.16, 22.75)
  point P27 (-2.7, 25.25)
  point P28 (-2.7, 22.75)
  point P29 (-5.24, 25.25)
  point P30 (-5.24, 22.75)
  point P31 (-7.78, 25.25)
  point P32 (-7.78, 22.75)
  point P33 (-10.32, 25.25)
  point P34 (-10.32, 22.75)
  point P35 (-12.86, 25.25)
  point P36 (-12.86, 22.75)
  point P37 (-15.4, 25.25)
  point P38 (-15.4, 22.75)
  point P39 (-17.94, 25.25)
  point P40 (-17.94, 22.75)
  point P41 (-20.48, 25.25)
  point P42 (-20.48, 22.75)
  point P43 (-23.02, 25.25)
  point P44 (-23.02, 22.75)
  point P45 (-25.56, 25.25)
  point P46 (-25.56, 22.75)
  point P47 (-28.1, 25.25)
  point P48 (-28.1, 22.75)
  point P49 (25.24, -25.25)
  point P50 (22.7, -25.25)
  point P51 (20.16, -25.25)
  point P52 (17.62, -25.25)
  point P53 (15.08, -25.25)
  point P54 (12.54, -25.25)
  point P55 (10, -25.25)
  point P56 (7.46, -25.25)
  point P57 (4.92, -25.25)
  point P58 (2.38, -25.25)
  point P59 (-0.16, -25.25)
  point P60 (-2.7, -25.25)
  point P61 (-5.24, -25.25)
  point P62 (-7.78, -25.25)
  point P63 (-10.32, -25.25)
  point P64 (-12.86, -25.25)
  point P65 (-15.4, -25.25)
  point P66 (-17.94, -25.25)
  point P67 (-20.48, -25.25)
  point P68 (-23.02, -25.25)
  point P69 (-25.56, -25.25)
  point P70 (-28.1, -25.25)
  dimension "d18" = 58.8
  dimension "d19" = 5
  dimension "d20" = 2.5
  dimension "d22" = 1.2
  dimension "d23" = 1.2
  dimension "d26" = -2.54
  dimension "d27" = 0
  dimension "d28" = 2.5
  dimension "d32" = 18
  dimension "d33" = 10.8
  dimension "d44" = -0.4
  dimension "d47" = -2.54
  dimension "d48" = 0
  dimension "d49" = -0.4
  dimension "d52" = -2.54
  dimension "d53" = 0
  constraint horizontal L8
  constraint vertical L9
  constraint horizontal L10
  constraint vertical L11
  constraint midpoint L11 L12.start
  constraint midpoint L9 L12.end
  constraint horizontal L14
  constraint perpendicular L14 L15
  constraint parallel L14 L16
  constraint parallel L15 L17
  constraint coincident L18 P0
  constraint coincident L19 P0
  constraint symmetric L12 L14.start L22.end
  constraint symmetric L12 L14.end L21.start
  constraint symmetric L12 L15.end L20.start
  constraint symmetric L12 L16.end L20.end
  constraint parallel L201 L203
  constraint concentric A1 A4
  constraint concentric A0 A5
  constraint tangent A4 L200
  constraint tangent L200 A5
  constraint perpendicular L202 L204
  constraint perpendicular L204 L205
  constraint perpendicular L292 L375
  constraint perpendicular L282 L376
  constraint perpendicular L299 L377
  constraint perpendicular L290 L378
  constraint perpendicular L359 L379
  constraint perpendicular L366 L380
  constraint perpendicular L352 L381
  constraint perpendicular L271 L382
  constraint perpendicular L279 L383
  constraint perpendicular L283 L384
  constraint perpendicular L265 L385
  constraint perpendicular L267 L386
  constraint perpendicular L331 L387
  constraint perpendicular L334 L388
  constraint perpendicular L288 L389
  constraint perpendicular L259 L390
  constraint perpendicular L262 L391
  constraint perpendicular L260 L392
  constraint perpendicular L345 L393
  constraint perpendicular L217 L394
  constraint perpendicular L208 L395
  constraint perpendicular L208 L396
  constraint coincident P3 L401.start
  constraint perpendicular L394 L401
  constraint symmetric P2 L401 P4
  constraint symmetric L397.start L401 L403.start
  constraint symmetric L397.end L401 L402.start
  constraint symmetric L398.end L401 L402.end
  constraint symmetric L399.end L401 L404.start
  constraint symmetric L12 L582.start L586.end
  constraint symmetric L12 L582.end L587.end
  constraint symmetric L12 L583.end L588.end
  constraint symmetric L12 L584.end L586.start
  measures "d18" distance of L8.start L8.end
  measures "d19" distance of L8.start L10.end
  measures "d20" diameter of A2
  measures "d22" distance of L15.end L16.end
  measures "d23" distance of L14.end L15.end
  measures "d28" diameter of A3
  measures "d32" distance of L202.end L204.end
  measures "d33" distance of L204.end L205.end
extrude "Extrude2" add sketch "Sketch2" along normal blind 8 contours L8 L9 L11 L12 L13 | L9 L10 L11 L12 | L207 L209 L217 L394 bodies 1
extrude "Extrude3" add sketch "Sketch2" along normal blind 1.5 from surface at 4.5 separate body contours A4 L200 A5 L201 L202 L203 L204 L205 L208 L395 L396 makes body 2
extrude "Extrude4" cut sketch "Sketch2" against normal through all contours A2 | A3 | A6 | A7 bodies 1
sketch "Sketch3" plane through (0, 0, 1.67) normal (0, 0, 1) x (-1, 0, 0)
  circle A0 centre (33.25, -22.5) radius 1.25
  circle A1 centre (-32.75, -24) radius 1.25
  circle A2 centre (33.25, 22.5) radius 1.25
  circle A3 centre (-32.75, 24) radius 1.25
  arc A4 (38.25, 17.5) -> (28.25, 27.5) centre (28.25, 17.5) ccw
  line L0 (28.25, 27.5) -> (-38.25, 27.5)
  line L1 (-38.25, 27.5) -> (-38.25, 12.5)
  line L2 (-38.25, 12.5) -> (-26.25, 12.5)
  line L3 (-26.25, 12.5) -> (-26.25, -7.5)
  line L4 (-26.25, -7.5) -> (-35.75, -7.5)
  line L5 (-35.75, -7.5) -> (-35.75, -27.5)
  line L6 (-35.75, -27.5) -> (28.25, -27.5)
  arc A5 (28.25, -27.5) -> (38.25, -17.5) centre (28.25, -17.5) ccw
  line L7 (38.25, -17.5) -> (38.25, 17.5)
  line L8 (32, -23.2217) -> (33.25, -23.9434)
  line L9 (33.25, -23.9434) -> (34.5, -23.2217)
  line L10 (34.5, -23.2217) -> (34.5, -21.7783)
  line L11 (34.5, -21.7783) -> (33.25, -21.0566)
  line L12 (33.25, -21.0566) -> (32, -21.7783)
  line L13 (32, -21.7783) -> (32, -23.2217)
  line L14 (32, 21.7783) -> (33.25, 21.0566)
  line L15 (33.25, 21.0566) -> (34.5, 21.7783)
  line L16 (34.5, 21.7783) -> (34.5, 23.2217)
  line L17 (34.5, 23.2217) -> (33.25, 23.9434)
  line L18 (33.25, 23.9434) -> (32, 23.2217)
  line L19 (32, 23.2217) -> (32, 21.7783)
  line L20 (33.25, -25.0981) -> (35.5, -23.799)
  line L21 (35.5, -23.799) -> (35.5, -21.201)
  line L22 (35.5, -21.201) -> (33.25, -19.9019)
  line L23 (33.25, -19.9019) -> (31, -21.201)
  line L24 (31, -21.201) -> (31, -23.799)
  line L25 (31, -23.799) -> (33.25, -25.0981)
  line L26 (33.25, 19.9019) -> (35.5, 21.201)
  line L27 (35.5, 21.201) -> (35.5, 23.799)
  line L28 (35.5, 23.799) -> (33.25, 25.0981)
  line L29 (33.25, 25.0981) -> (31, 23.799)
  line L30 (31, 23.799) -> (31, 21.201)
  line L31 (31, 21.201) -> (33.25, 19.9019)
  line L32 (29.05, -21.5) -> (29.05, -26.5)
  line L33 (29.05, -26.5) -> (-29.75, -26.5)
  line L34 (-29.75, -26.5) -> (-29.75, -21.5)
  line L35 (-29.75, -21.5) -> (29.05, -21.5)
  line L36 (-29.75, 21.5) -> (-29.75, 26.5)
  line L37 (-29.75, 26.5) -> (29.05, 26.5)
  line L38 (29.05, 26.5) -> (29.05, 21.5)
  line L39 (29.05, 21.5) -> (-29.75, 21.5)
  point P0 (33.25, -22.5)
  point P1 (33.25, 22.5)
  dimension "d40" = 1
  dimension "d41" = 1
  constraint coincident P0 A0.centre
  constraint coincident P1 A2.centre
extrude "Extrude5" add sketch "Sketch3" along normal up to surface (4.5 mm away) contours L20 L21 L22 L23 L24 L25 | L26 L27 L28 L29 L30 L31 bodies 1 2
sketch "Sketch4" plane through (0, 0, 0) normal (0, 0, -1) x (1, 0, 0)
  circle A0 centre (-33.25, -22.5) radius 1.25
  circle A1 centre (32.75, -24) radius 1.25
  circle A2 centre (-33.25, 22.5) radius 1.25
  circle A3 centre (32.75, 24) radius 1.25
  arc A4 (-28.25, 27.5) -> (-38.25, 17.5) centre (-28.25, 17.5) ccw
  line L0 (-38.25, 17.5) -> (-38.25, -17.5)
  arc A5 (-38.25, -17.5) -> (-28.25, -27.5) centre (-28.25, -17.5) ccw
  line L1 (-28.25, -27.5) -> (35.75, -27.5)
  line L2 (35.75, -27.5) -> (35.75, -7.5)
  line L3 (35.75, -7.5) -> (26.25, -7.5)
  line L4 (26.25, -7.5) -> (26.25, 12.5)
  line L5 (26.25, 12.5) -> (38.25, 12.5)
  line L6 (38.25, 12.5) -> (38.25, 27.5)
  line L7 (38.25, 27.5) -> (-28.25, 27.5)
  line L8 (-32.5283, 21.25) -> (-31.8066, 22.5)
  line L9 (-31.8066, 22.5) -> (-32.5283, 23.75)
  line L10 (-32.5283, 23.75) -> (-33.9717, 23.75)
  line L11 (-33.9717, 23.75) -> (-34.6934, 22.5)
  line L12 (-34.6934, 22.5) -> (-33.9717, 21.25)
  line L13 (-33.9717, 21.25) -> (-32.5283, 21.25)
  line L14 (33.4717, 22.75) -> (34.1934, 24)
  line L15 (34.1934, 24) -> (33.4717, 25.25)
  line L16 (33.4717, 25.25) -> (32.0283, 25.25)
  line L17 (32.0283, 25.25) -> (31.3066, 24)
  line L18 (31.3066, 24) -> (32.0283, 22.75)
  line L19 (32.0283, 22.75) -> (33.4717, 22.75)
  line L20 (33.4717, -25.25) -> (34.1934, -24)
  line L21 (34.1934, -24) -> (33.4717, -22.75)
  line L22 (33.4717, -22.75) -> (32.0283, -22.75)
  line L23 (32.0283, -22.75) -> (31.3066, -24)
  line L24 (31.3066, -24) -> (32.0283, -25.25)
  line L25 (32.0283, -25.25) -> (33.4717, -25.25)
  line L26 (-32.5513, -23.763) -> (-31.8069, -22.5264)
  line L27 (-31.8069, -22.5264) -> (-32.5055, -21.2634)
  line L28 (-32.5055, -21.2634) -> (-33.9487, -21.237)
  line L29 (-33.9487, -21.237) -> (-34.6931, -22.4736)
  line L30 (-34.6931, -22.4736) -> (-33.9945, -23.7366)
  line L31 (-33.9945, -23.7366) -> (-32.5513, -23.763)
  line L32 (-34.549, 24.75) -> (-35.8481, 22.5)
  line L33 (-35.8481, 22.5) -> (-34.549, 20.25)
  line L34 (-34.549, 20.25) -> (-31.951, 20.25)
  line L35 (-31.951, 20.25) -> (-30.6519, 22.5)
  line L36 (-30.6519, 22.5) -> (-31.951, 24.75)
  line L37 (-31.951, 24.75) -> (-34.549, 24.75)
  line L38 (-34.5076, -20.2266) -> (-35.8476, -22.4524)
  line L39 (-35.8476, -22.4524) -> (-34.59, -24.7258)
  line L40 (-34.59, -24.7258) -> (-31.9924, -24.7734)
  line L41 (-31.9924, -24.7734) -> (-30.6524, -22.5476)
  line L42 (-30.6524, -22.5476) -> (-31.91, -20.2742)
  line L43 (-31.91, -20.2742) -> (-34.5076, -20.2266)
  line L44 (34.049, -21.75) -> (31.451, -21.75)
  line L45 (31.451, -21.75) -> (30.1519, -24)
  line L46 (30.1519, -24) -> (31.451, -26.25)
  line L47 (31.451, -26.25) -> (34.049, -26.25)
  line L48 (34.049, -26.25) -> (35.3481, -24)
  line L49 (35.3481, -24) -> (34.049, -21.75)
  line L50 (31.451, 26.25) -> (30.1519, 24)
  line L51 (30.1519, 24) -> (31.451, 21.75)
  line L52 (31.451, 21.75) -> (34.049, 21.75)
  line L53 (34.049, 21.75) -> (35.3481, 24)
  line L54 (35.3481, 24) -> (34.049, 26.25)
  line L55 (34.049, 26.25) -> (31.451, 26.25)
  point P0 (-33.25, 22.5)
  point P1 (-33.25, -22.5)
  point P2 (32.75, 24)
  point P3 (32.75, -24)
  point P4 (-33.25, -22.5)
  dimension "d56" = 1
  dimension "d57" = 1
  dimension "d58" = 1
  dimension "d59" = 1
  constraint coincident P0 A2.centre
  constraint coincident P4 A0.centre
  constraint coincident P2 A3.centre
  constraint coincident P3 A1.centre
extrude "Extrude6" [suppressed]
extrude "Extrude7" [suppressed]
move_body "Move1" [suppressed]
move_body "Move2" [suppressed]
move_body "Move3" [suppressed]
